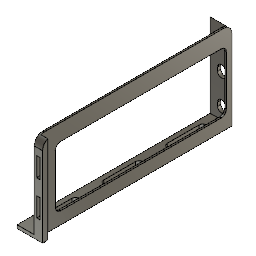
GPU_mount (Autodesk Fusion 360 design; units mm, degrees)
Autodesk Fusion 360 part; units mm, degrees
mesh "Mesh1" [no effect]
sketch "Sketch1" plane through (0, 0, 0) normal (0, 1, 0) x (1, 0, 0)
  line L0 (11.7684, -30.12) -> (12.655, -30.12) construction
  line L1 (12.655, -30.12) -> (12.655, -40.3647) construction
  line L2 (12.655, -40.3647) -> (11.7684, -40.3647) construction
  line L3 (11.7684, -40.3647) -> (11.7684, -30.12) construction
  line L4 (11.7684, -9.7924) -> (12.655, -9.7924) construction
  line L5 (12.655, -9.7924) -> (12.655, -19.9878) construction
  line L6 (12.655, -19.9878) -> (11.7684, -19.9878) construction
  line L7 (11.7684, -19.9878) -> (11.7684, -9.7924) construction
  line L8 (11.2684, -9.2924) -> (13.155, -9.2924)
  line L9 (13.155, -9.2924) -> (13.155, -20.4878)
  line L10 (13.155, -20.4878) -> (11.2684, -20.4878)
  line L11 (11.2684, -20.4878) -> (11.2684, -9.2924)
  line L12 (13.155, -40.8647) -> (11.2684, -40.8647)
  line L13 (11.2684, -40.8647) -> (11.2684, -29.62)
  line L14 (11.2684, -29.62) -> (13.155, -29.62)
  line L15 (13.155, -29.62) -> (13.155, -40.8647)
  line L16 (12.2117, -40.3647) -> (12.2117, -9.7924) construction
  line L17 (14.7117, -0.0785) -> (9.7117, -0.0785)
  line L18 (9.7117, -0.0785) -> (9.7117, -50.0785)
  line L19 (9.7117, -50.0785) -> (14.7117, -50.0785)
  line L20 (14.7117, -50.0785) -> (14.7117, -0.0785)
  line L21 (14.7117, -0.0785) -> (9.7117, -50.0785) construction
  line L22 (9.7117, -0.0785) -> (14.7117, -50.0785) construction
  line L23 (10.7117, -50.0785) -> (10.7117, -0.0785)
  line L24 (6.4117, -5.7839) -> (6.4117, -25.7839) construction
  circle A0 centre (6.4117, -25.7839) radius 2.25
  circle A1 centre (6.4117, -5.7839) radius 2.25
  circle A2 centre (6.4117, -8.0339) radius 2.25
  circle A3 centre (6.4117, -23.5339) radius 2.25
  line L25 (4.1617, -23.5339) -> (4.1617, -25.7839)
  line L26 (8.6617, -25.7839) -> (8.6617, -23.5339)
  line L27 (4.1617, -8.0339) -> (4.1617, -5.7839)
  line L28 (8.6617, -5.7839) -> (8.6617, -8.0339)
  line L29 (10.7117, -0.0785) -> (14.7117, -0.0785)
  line L30 (14.7117, -0.0785) -> (14.7117, 1.9215)
  line L31 (14.7117, 1.9215) -> (10.7117, 1.9215)
  line L32 (10.7117, 1.9215) -> (10.7117, -0.0785)
  point P0 (12.2117, -25.0785)
  point P1 (12.2117, -25.0785)
  dimension "d1" = -0.5
  dimension "d2" = -0.5
  dimension "d3" = 5
  dimension "d13" = 50
  dimension "d19" = 3.3
  dimension "d20" = 20
  dimension "d21" = 4.5
  dimension "d22" = 4.5
  dimension "d31" = 1
  dimension "d39" = 4.5
  dimension "d40" = 4.5
  dimension "d44" = 2
  constraint horizontal L0
  constraint vertical L1
  constraint horizontal L2
  constraint vertical L3
  constraint horizontal L4
  constraint vertical L5
  constraint horizontal L6
  constraint vertical L7
  constraint midpoint L2 L16.start
  constraint midpoint L4 L16.end
  constraint midpoint L16 P1
  constraint perpendicular L17 L18
  constraint parallel L17 L19
  constraint parallel L18 L20
  constraint horizontal L17
  constraint coincident L21 P1
  constraint coincident L22 P1
  constraint coincident P1 P0
  constraint coincident L19 L23.start
  constraint coincident L17 L23.end
  constraint perpendicular L17 L23
  constraint parallel L18 L24
  constraint coincident L24.end A0.centre
  constraint coincident L24.start A1.centre
  constraint coincident L24 A2.centre
  constraint coincident A1 A2.centre
  constraint coincident A0 A3.centre
  constraint coincident L24 A3.centre
  constraint coincident A3 L25.start
  constraint coincident A0 L25.end
  constraint tangent A0 L25
  constraint parallel L24 L25
  constraint coincident A0 L26.start
  constraint coincident A3 L26.end
  constraint tangent A3 L26
  constraint parallel L24 L26
  constraint coincident A2 L27.start
  constraint coincident A1 L27.end
  constraint tangent A1 L27
  constraint parallel L26 L27
  constraint coincident A1 L28.start
  constraint coincident A2 L28.end
  constraint tangent A2 L28
  constraint parallel L27 L28
  constraint horizontal L29
  constraint vertical L30
  constraint horizontal L31
  constraint vertical L32
  measures "d3" distance of L18.end L19.end
  measures "d13" distance of L17 L19
  measures "d19" distance of L18 L24
  measures "d20" distance of L24.start L24.end
  measures "d21" diameter of A0
  measures "d22" diameter of A1
  measures "d31" distance of L18 L23
  measures "d39" diameter of A2
  measures "d40" diameter of A3
  measures "d44" distance of L23.end L31.end
extrude "Extrude1" add sketch "Sketch1" along normal blind 3 from surface at -19 contours L17 L19 L20 L23 L29 | L17 L18 L19 L23
extrude "Extrude2" add sketch "Sketch1" along normal blind 96 and the other way blind 16 contours L17 L18 L19 L23
sketch "Sketch2" plane through (9.7117, 0, 0) normal (-1, 0, 0) x (0, -1, 0)
  line L0 (19, 0.0785) -> (19, 50.0785)
  line L1 (19, 50.0785) -> (-96, 50.0785)
  line L2 (-96, 50.0785) -> (-96, 0.0785)
  line L3 (-96, 0.0785) -> (19, 0.0785)
  line L4 (-94, 0.0785) -> (-94, 50.0785)
  line L5 (-89.58, 5.3807) -> (4.42, 5.3807)
  line L6 (7.42, 8.3807) -> (7.42, 37.3807)
  line L7 (4.42, 40.3807) -> (-89.58, 40.3807)
  line L8 (-92.58, 37.3807) -> (-92.58, 8.3807)
  line L9 (-96, 0.0785) -> (19, 0.0785)
  line L10 (19, 0.0785) -> (19, -1.9215)
  line L11 (19, -1.9215) -> (-96, -1.9215)
  line L12 (-96, -1.9215) -> (-96, 0.0785)
  arc A0 (-92.58, 8.3807) -> (-89.58, 5.3807) centre (-89.58, 8.3807) ccw
  arc A1 (-89.58, 40.3807) -> (-92.58, 37.3807) centre (-89.58, 37.3807) ccw
  arc A2 (7.42, 37.3807) -> (4.42, 40.3807) centre (4.42, 37.3807) ccw
  arc A3 (4.42, 5.3807) -> (7.42, 8.3807) centre (4.42, 8.3807) ccw
  dimension "d14" = 2
  dimension "d26" = 2
  dimension "d41" = 3
  dimension "d42" = 35
  dimension "d43" = 100
  constraint coincident L3 L4.start
  constraint coincident L1 L4.end
  constraint perpendicular L1 L4
  constraint horizontal L5
  constraint vertical L6
  constraint horizontal L7
  constraint vertical L8
  constraint horizontal L9
  constraint vertical L10
  constraint horizontal L11
  constraint vertical L12
  constraint coincident L2.end L3.start
  constraint tangent L5 A0
  constraint tangent L8 A0
  constraint tangent L7 A1
  constraint tangent L8 A1
  constraint equal A0 A1
  constraint tangent L6 A2
  constraint tangent L7 A2
  constraint equal A0 A2
  constraint tangent L5 A3
  constraint tangent L6 A3
  constraint equal A0 A3
  measures "d14" distance of L2 L4
  measures "d26" distance of L2.end L11.end
  measures "d41" radius of A0
  measures "d42" distance of L5 L7
  measures "d43" distance of L6 L8
extrude "Extrude3" cut sketch "Sketch2" against normal blind 10 contours L5 L6 L7 L8 A0 A1 A2 A3
extrude "Extrude4" add sketch "Sketch2" along normal blind 10 contours L1 L2 L3 L4 L9
extrude "Extrude5" cut sketch "Sketch1" along normal blind 190 contours A0 A3 | A0 A3 L25 | A0 A3 L26 | A0 A3 | A0 A3 | A1 A2 | A1 A2 L28 | A1 A2 L27 | A1 A2 | A1 A2
extrude "Extrude6" add sketch "Sketch2" along normal blind 10 and the other way blind 1 contours L3 L9 L10 L11 L12
sketch "Sketch3" plane through (0, 0, 0.0785) normal (0, 0, 1) x (-1, 0, 0)
  line L0 (-9.7117, 19) -> (-9.7117, -94)
  line L1 (-9.7117, -94) -> (0.2883, -94)
  line L2 (0.2883, -94) -> (0.2883, 19)
  line L3 (0.2883, 19) -> (-9.7117, 19)
  line L4 (-4.7117, -94) -> (-4.7117, 19) construction
  circle A0 centre (-4.7117, 8.1673) radius 2.25
  circle A1 centre (-4.7117, -10.4327) radius 2.25
  circle A2 centre (-4.7117, -29.0327) radius 2.25
  circle A3 centre (-4.7117, -47.6327) radius 2.25
  circle A4 centre (-4.7117, -66.2327) radius 2.25
  circle A5 centre (-4.7117, -84.8327) radius 2.25
  line L5 (-2.4617, -84.8327) -> (-2.4617, -66.2327)
  line L6 (-6.9617, -66.2327) -> (-6.9617, -84.8327)
  line L7 (-2.4617, -47.6327) -> (-2.4617, -29.0327)
  line L8 (-6.9617, -47.6327) -> (-6.9617, -29.0327)
  line L9 (-2.4617, -10.4327) -> (-2.4617, 8.1673)
  line L10 (-6.9617, 8.1673) -> (-6.9617, -10.4327)
  dimension "d32" = 4.5
  dimension "d35" = 0
  dimension "d36" = -93
  constraint midpoint L1 L4.start
  constraint midpoint L3 L4.end
  constraint coincident L4 A0.centre
  constraint coincident A5 L5.start
  constraint coincident A4 L5.end
  constraint tangent A4 L5
  constraint parallel L4 L5
  constraint coincident A4 L6.start
  constraint coincident A5 L6.end
  constraint tangent A5 L6
  constraint parallel L4 L6
  constraint coincident A3 L7.start
  constraint coincident A2 L7.end
  constraint tangent A2 L7
  constraint parallel L4 L7
  constraint coincident A3 L8.start
  constraint coincident A2 L8.end
  constraint tangent A2 L8
  constraint parallel L4 L8
  constraint coincident A1 L9.start
  constraint coincident A0 L9.end
  constraint tangent A0 L9
  constraint parallel L8 L9
  constraint coincident A0 L10.start
  constraint coincident A1 L10.end
  constraint tangent A1 L10
  constraint parallel L4 L10
  measures "d32" diameter of A0
extrude "Extrude7" cut sketch "Sketch3" against normal blind 10 contours A0 | A0 A1 L9 L10 | A1 | A2 | A2 A3 L7 L8 | A3 | A4 | A4 A5 L5 L6 | A5
extrude "Extrude8" add sketch "Sketch1" along normal blind 3 from surface at -19 contours L17 L29 L30 L31 L32
fillet "Fillet1" radius 5 2 edges at (12.2117, -19, 50.0785) (5.2117, 96, 50.0785)
named bodies: "GPU_front"
